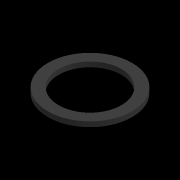
# Autodesk Inventor part: pg7_gasket
Saved by Autodesk Inventor 2020.2 (Build 242310000, 310)
## iProperties
Created: 2020-04-23
Part Number: pg7_gasket
Material: Rubber, Silicone
Document SubType Name: Modeling
Designer: agmlego
Mass: 0.122044 g
Surface Area: 2.87161 cm^2
Volume: 0.0976348 cm^3
Density: 1.25 g/cm^3
Appearance: Rubber - Black
Author: agmlego
Autodesk Inventor part; units mm, degrees
ref_plane "YZ Plane" through (0, 0, 0) normal (1, 0, 0) x (0, 1, 0)
ref_plane "XZ Plane" through (0, 0, 0) normal (0, 1, 0) x (-1, 0, 0)
ref_plane "XY Plane" through (0, 0, 0) normal (0, 0, 1) x (1, 0, 0)
sketch "Sketch1" plane through (0, 0, 0) normal (0, 1, 0) x (-1, 0, 0)
  circle A0 centre (0, 0) radius 8.375
  circle A1 centre (0, 0) radius 6.25
  dimension "d0" = 16.75
  dimension "d1" = 12.5
  constraints: 2 centre point, 2 coincident
  measures "d0" diameter of A0
  measures "d1" diameter of A1
extrude "Extrusion1" add sketch "Sketch1" along normal blind 1
body "Solid1"
